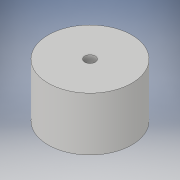
# Autodesk Inventor part: roller2 grp17
Saved by Autodesk Inventor 2019 (Build 230136000, 136)
## iProperties
Created: 2020-02-17
Part Number: roller2 grp17
Material: Generic
Document SubType Name: Modeling
Designer: Aishwarya
Density: 1 g/cm^3
Appearance: Default
Author: Aishwarya
Autodesk Inventor part; units mm, degrees
ref_plane "YZ Plane" through (0, 0, 0) normal (1, 0, 0) x (0, 1, 0)
ref_plane "XZ Plane" through (0, 0, 0) normal (0, 1, 0) x (-1, 0, 0)
ref_plane "XY Plane" through (0, 0, 0) normal (0, 0, 1) x (1, 0, 0)
sketch "Sketch1" plane through (0, 0, 0) normal (0, 1, 0) x (-1, 0, 0)
  circle A0 centre (0, 0) radius 17.5
  circle A1 centre (0, 0) radius 2.5
  dimension "d0" = 35
  dimension "d1" = 5
  constraints: 2 centre point, 2 coincident
  measures "d0" diameter of A0
  measures "d1" diameter of A1
extrude "Extrusion1" add sketch "Sketch1" against normal blind 25
thicken "Thicken1" operation add thickness 1 both sides no extend neighbours yes toward (-0.9967573, 0, -0.0804666) faces at (-17.4433, -16.6667, -1.4082)
thicken "Thicken2" operation add thickness 1 both sides no extend neighbours yes toward (-0.9967573, 0, -0.0804666) faces at (-18.44, -16.6667, -1.4886)
body "Solid1"
